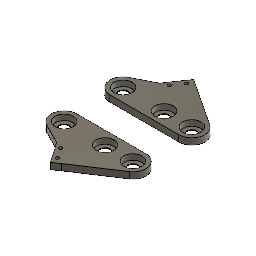
Side Arms v8 (Autodesk Fusion 360 design; units mm, degrees)
Autodesk Fusion 360 part; units mm, degrees
note: some values were not read from the file. Set by a fixed rule: which sketch regions a step uses.
sketch "Sketch1" plane through (0, 0, 0) normal (0, 1, 0) x (1, 0, 0)
  circle A0 centre (0, 0) radius 11
  circle A1 centre (0, 0) radius 16
  line L0 (0, 0) -> (-34, 0)
  circle A2 centre (-34, 0) radius 11
  circle A3 centre (-34, 0) radius 16
  line L1 (-34, 0) -> (-84, 0)
  circle A4 centre (-84, 0) radius 11
  circle A5 centre (-84, 0) radius 16
  circle A6 centre (-84, 0) radius 27.5
  circle A7 centre (0, 0) radius 56.5
  circle A8 centre (0, 0) radius 71.5
  line L2 (-84, 16) -> (0, 16)
  circle A9 centre (-34, 0) radius 6
  circle A10 centre (0, 0) radius 6
  circle A11 centre (-84, 0) radius 6
  line L3 (-66.2029, -27.0078) -> (-49.2957, -51.7898)
  line L4 (-49.2957, -51.7898) -> (-41.0351, -46.154)
  line L5 (-41.0351, -46.154) -> (-57.9423, -21.372)
  line L6 (-57.9423, -21.372) -> (-66.2029, -27.0078)
  line L7 (-41.0351, -46.154) -> (8.7948, -13.366)
  line L8 (-66.2029, -27.0078) -> (-91.2559, -14.2601)
  line L9 (-45.1654, -48.9719) -> (-62.0726, -24.1899)
  line L10 (-57.7493, -39.3988) -> (-49.4887, -33.763)
  line L11 (-49.2957, -51.7898) -> (-49.4887, -33.763)
  line L12 (-66.2029, -27.0078) -> (-49.4887, -33.763)
  circle A12 centre (-57.8458, -30.3854) radius 2
  circle A13 centre (-49.3922, -42.7764) radius 2
  point P0 (-66.2029, -27.0078)
  dimension "d1" = 22
  dimension "d2" = 32
  dimension "d3" = 34
  dimension "d4" = 22
  dimension "d5" = 32
  dimension "d8" = 50
  dimension "d10" = 22
  dimension "d11" = 32
  dimension "d12" = 55
  dimension "d14" = 143
  dimension "d17" = 113
  dimension "d31" = 12
  dimension "d32" = 12
  dimension "d33" = 12
  dimension "d42" = 30
  dimension "d43" = 10
  dimension "d44" = 4
  dimension "d45" = 4
  constraint coincident A0.centre A1.centre
  constraint horizontal L0
  constraint coincident L0.end A2.centre
  constraint concentric A2 A3
  constraint parallel L0 L1
  constraint concentric A4 A5
  constraint concentric A4 A6
  constraint tangent A6 A7
  constraint concentric A0 A8
  constraint coincident A5 L2.start
  constraint coincident A1 L2.end
  constraint tangent A1 L2
  constraint tangent A5 L2
  constraint concentric A4 A11
  constraint perpendicular L3 L4
  constraint parallel L3 L5
  constraint parallel L4 L6
  constraint coincident A8 L3.end
  constraint coincident P0 L3.start
  constraint coincident A1 L7.end
  constraint tangent A1 L7
  constraint coincident A5 L8.end
  constraint tangent A5 L8
  constraint midpoint L4 L9.start
  constraint midpoint L6 L9.end
  constraint midpoint L3 L10.start
  constraint midpoint L5 L10.end
  constraint midpoint L12 A12.centre
  constraint midpoint L11 A13.centre
  measures "d1" diameter of A0
  measures "d2" diameter of A1
  measures "d3" distance of A0.centre L0.end
  measures "d4" diameter of A2
  measures "d5" diameter of A3
  measures "d8" distance of L0.end L1.end
  measures "d10" diameter of A4
  measures "d11" diameter of A5
  measures "d12" diameter of A6
  measures "d14" diameter of A8
  measures "d17" diameter of A7
  measures "d31" diameter of A9
  measures "d32" diameter of A10
  measures "d33" diameter of A11
  measures "d42" distance of P0 L3.end
  measures "d43" distance of P0 L5.end A0
  measures "d44" diameter of A12
  measures "d45" diameter of A13
extrude "Extrude1" [suppressed]
extrude "Extrude2" [suppressed]
extrude "Extrude3" [suppressed]
extrude "Extrude4" [suppressed]
extrude "Extrude5" [suppressed]
extrude "Extrude6" [suppressed]
chamfer "Chamfer1" [suppressed]
extrude "Extrude7" add sketch "Sketch1" along normal blind 8 contours A1 | A1 L0 A3 L2 | A1 L0 A3 L1 A7 L7 | L0 A2 A3 L1 | A3 L1 A7 L2 | A6 A7 A8 L5 L6 L7 | L0 A2 A3 L1 | A6 A7 L2 | L1 A5 A6 A8 | L1 A5 A6 A8 L2 | L4 L5 L9 L11 A13 | L1 A5 A8 | L1 A5 A8 | A6 A8 L8 | A5 A6 A8 L8 | L4 L9 L11 A13 | L5 L6 L9 L12 A12 | L9 L10 L11 A13 | L9 L10 L12 A12 | A5 A8 L2 | A5 A8 | L3 L9 L10 L12 A12 | L6 L9 L12 A12 | L3 L9 L10 L11 A13 makes body 1
extrude "Extrude8" add sketch "Sketch1" along normal blind 1 contours A0 | L0 A2 L1 A9 | L0 A2 L1 A9 | A4 bodies 1
chamfer "Chamfer2" distance 2 angle 45 2 edges at (-59.7105, 8, 29.6622) (-51.2569, 8, 42.0532) on bodies 1
delete_face "DeleteFace1" 1 faces at (-50.6912, 7.5556, 46.0862) on bodies 1
delete_face "DeleteFace2" 1 faces at (-58.1115, 7.5556, 33.931) on bodies 1
chamfer "Chamfer3" distance 2 angle 45 2 edges at (-51.2569, 0, 42.0532) (-59.7105, 0, 29.6622) on bodies 1
ref_plane "WorkPlane2" through (-42, 4, -36) normal (0, 0, -1) x (-1, 0, 0)
mirror "Mirror1" about plane through (-42, 4, -36) normal (0, 0, -1) of bodies 1 makes body 2
